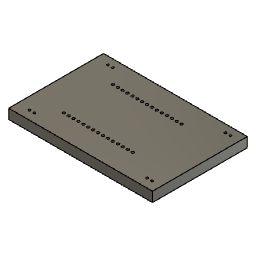
Rover base v1 (Autodesk Fusion 360 design; units mm, degrees)
Autodesk Fusion 360 part; units mm, degrees
sketch "Sketch1" plane through (0, 0, 0) normal (0, 1, 0) x (1, 0, 0)
  line L0 (6.0632, -5.8759) -> (64.7731, -5.8759)
  line L1 (64.7731, -5.8759) -> (64.7731, -44.5785)
  line L2 (64.7731, -44.5785) -> (6.0632, -44.5785)
  line L3 (6.0632, -44.5785) -> (6.0632, -5.8759)
  circle A0 centre (11, -9) radius 0.45
  circle A1 centre (13, -9) radius 0.45
  circle A2 centre (13, -41) radius 0.45
  circle A3 centre (11, -41) radius 0.45
  circle A4 centre (61, -9) radius 0.45
  circle A5 centre (59, -9) radius 0.45
  circle A6 centre (61, -41) radius 0.45
  circle A7 centre (59, -41) radius 0.45
  circle A8 centre (19, -15) radius 0.5
  circle A9 centre (21, -15) radius 0.5
  circle A10 centre (23, -15) radius 0.5
  circle A11 centre (25, -15) radius 0.5
  circle A12 centre (27, -15) radius 0.5
  circle A13 centre (29, -15) radius 0.5
  circle A14 centre (31, -15) radius 0.5
  circle A15 centre (33, -15) radius 0.5
  circle A16 centre (35, -15) radius 0.5
  circle A17 centre (37, -15) radius 0.5
  circle A18 centre (39, -15) radius 0.5
  circle A19 centre (41, -14.9013) radius 0.5
  circle A20 centre (43, -14.9013) radius 0.5
  circle A21 centre (45, -14.9013) radius 0.5
  circle A22 centre (47, -14.9013) radius 0.5
  circle A23 centre (25, -35) radius 0.5
  circle A24 centre (47, -34.9013) radius 0.5
  circle A25 centre (19, -35) radius 0.5
  circle A26 centre (29, -35) radius 0.5
  circle A27 centre (43, -34.9013) radius 0.5
  circle A28 centre (39, -35) radius 0.5
  circle A29 centre (37, -35) radius 0.5
  circle A30 centre (35, -35) radius 0.5
  circle A31 centre (33, -35) radius 0.5
  circle A32 centre (45, -34.9013) radius 0.5
  circle A33 centre (27, -35) radius 0.5
  circle A34 centre (23, -35) radius 0.5
  circle A35 centre (31, -35) radius 0.5
  circle A36 centre (41, -34.9013) radius 0.5
  circle A37 centre (21, -35) radius 0.5
  dimension "d1" = 0.9
  dimension "d2" = 0.9
  dimension "d3" = 0.9
  dimension "d4" = 0.9
  dimension "d5" = 0.9
  dimension "d6" = 0.9
  dimension "d7" = 0.9
  dimension "d8" = 0.9
  dimension "d28" = 1
  dimension "d29" = 1
  dimension "d30" = 1
  dimension "d31" = 1
  dimension "d32" = 1
  dimension "d33" = 1
  dimension "d34" = 1
  dimension "d35" = 1
  dimension "d36" = 1
  dimension "d37" = 1
  dimension "d38" = 1
  dimension "d39" = 1
  dimension "d40" = 1
  dimension "d41" = 1
  dimension "d42" = 1
  dimension "d43" = 1
  dimension "d44" = 1
  dimension "d45" = 1
  dimension "d46" = 1
  dimension "d47" = 1
  dimension "d48" = 1
  dimension "d49" = 1
  dimension "d50" = 1
  dimension "d51" = 1
  dimension "d52" = 1
  dimension "d53" = 1
  dimension "d54" = 1
  dimension "d55" = 1
  dimension "d56" = 1
  dimension "d57" = 1
  constraint horizontal L0
  constraint vertical L1
  constraint horizontal L2
  constraint vertical L3
  measures "d1" diameter of A0
  measures "d2" diameter of A1
  measures "d3" diameter of A3
  measures "d4" diameter of A2
  measures "d5" diameter of A5
  measures "d6" diameter of A4
  measures "d7" diameter of A7
  measures "d8" diameter of A6
  measures "d28" diameter of A8
  measures "d29" diameter of A9
  measures "d30" diameter of A10
  measures "d31" diameter of A11
  measures "d32" diameter of A12
  measures "d33" diameter of A13
  measures "d34" diameter of A14
  measures "d35" diameter of A15
  measures "d36" diameter of A16
  measures "d37" diameter of A17
  measures "d38" diameter of A18 A6.centre
  measures "d39" diameter of A19
  measures "d40" diameter of A20
  measures "d41" diameter of A21
  measures "d42" diameter of A22
  measures "d43" diameter of A25
  measures "d44" diameter of A37
  measures "d45" diameter of A34
  measures "d46" diameter of A23
  measures "d47" diameter of A33
  measures "d48" diameter of A26
  measures "d49" diameter of A35
  measures "d50" diameter of A31
  measures "d51" diameter of A30
  measures "d52" diameter of A29
  measures "d53" diameter of A28 A6.centre
  measures "d54" diameter of A36
  measures "d55" diameter of A27
  measures "d56" diameter of A32
  measures "d57" diameter of A24
extrude "Extrude1" add sketch "Sketch1" along normal blind 4
